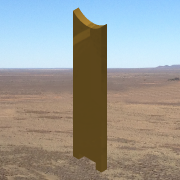
# Autodesk Inventor part: 2f1ar
Saved by Autodesk Inventor 2013 SP2 (Build 170200200, 200)
## iProperties
Company: HERA Project
Created: 2013-12-20
Part Number: 2f1ar
Material: Brass, Soft Yellow
Document SubType Name: Modeling
Designer: Rich Bradley
Mass: 28.2753 g
Surface Area: 26.7824 cm^2
Volume: 3.33829 cm^3
Density: 8.47 g/cm^3
Description: Feed arm pipe rest
Author: David DeBoer
Title: Dipole Arm Rest
Autodesk Inventor part; units mm, degrees
ref_plane "YZ Plane" through (0, 0, 0) normal (1, 0, 0) x (0, 1, 0)
ref_plane "XZ Plane" through (0, 0, 0) normal (0, 1, 0) x (-1, 0, 0)
ref_plane "XY Plane" through (0, 0, 0) normal (0, 0, 1) x (1, 0, 0)
sketch "Sketch1" plane through (0, 0, 0) normal (0, 0, 1) x (1, 0, 0)
  line L0 (0, 0) -> (15.875, 0)
  line L1 (15.875, 0) -> (15.875, 77.724)
  line L2 (15.875, 77.724) -> (0, 77.724)
  line L3 (0, 77.724) -> (0, 0)
  dimension "d0" = 77.724
  dimension "d1" = 15.875
  constraints: 8 end point, 2 parallel, 1 horizontal, 1 perpendicular
  measures "d0" distance of L2.end L0.start
  measures "d1" distance of L0.start L0.end
extrude "Extrusion1" add sketch "Sketch1" along normal blind 3.175
sketch "Sketch2" plane through (0, 0, 3.175) normal (0, 0, 1) x (1, 0, 0)
  line L0 (0, 0) -> (15.875, 0) projected
  line L1 (15.875, 77.724) -> (0, 77.724) projected
  line L2 (3.175, 0) -> (12.7, 0)
  line L3 (12.7, 0) -> (12.7, 3.175)
  line L4 (12.7, 3.175) -> (3.175, 3.175)
  line L5 (3.175, 3.175) -> (3.175, 0)
  line L6 (7.9375, 3.175) -> (7.9375, 0) construction
  line L7 (7.9375, 77.724) -> (7.9375, 0) construction
  dimension "d4" = 9.525
  dimension "d6" = 3.175
  constraints: 12 end point, 4 midpoint, 2 collinear, 2 parallel, 1 horizontal, 1 perpendicular
  measures "d4" distance of L3.end L4.end
  measures "d6" distance of L2.end L3.end
extrude "Extrusion2" cut sketch "Sketch2" against normal through all
sketch "Sketch3" plane through (0, 0, 3.175) normal (0, 0, 1) x (1, 0, 0)
  circle A0 centre (7.9375, 77.7875) radius 10.7315
  dimension "d11" = 21.463
  constraints: 1 centre point
  measures "d11" diameter of A0
extrude "Extrusion3" cut sketch "Sketch3" against normal blind 3.175
body "Solid1"
